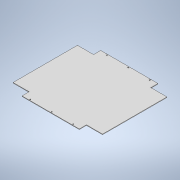
# Autodesk Inventor part: basePlate
Saved by Autodesk Inventor 2020 (Build 240168000, 168)
## iProperties
Created: 2019-06-20
Part Number: basePlate
Material: Generic
Document SubType Name: Modeling
Designer: Vivek Muskan
Density: 1 g/cm^3
Appearance: Default
Author: Vivek Muskan
Autodesk Inventor part; units mm, degrees
ref_plane "YZ Plane" through (0, 0, 0) normal (1, 0, 0) x (0, 1, 0)
ref_plane "XZ Plane" through (0, 0, 0) normal (0, 1, 0) x (-1, 0, 0)
ref_plane "XY Plane" through (0, 0, 0) normal (0, 0, 1) x (1, 0, 0)
sketch "Sketch1" plane through (0, 0, 0) normal (0, 1, 0) x (-1, 0, 0)
  line L0 (125, 90) -> (-125, 90)
  line L1 (-125, 90) -> (-125, -90)
  line L2 (-125, -90) -> (125, -90)
  line L3 (125, -90) -> (125, 90)
  line L4 (125, 90) -> (-125, -90) construction
  line L5 (-125, 90) -> (125, -90) construction
  line L6 (0, 90) -> (80, 90)
  line L7 (80, 90) -> (-80, 90)
  line L8 (-80, 90) -> (-80, 110)
  line L9 (-80, 110) -> (80, 110)
  line L10 (80, 110) -> (80, 90)
  line L11 (80, -90) -> (-80, -90)
  line L12 (-80, -90) -> (-80, -110)
  line L13 (-80, -110) -> (80, -110)
  line L14 (80, -110) -> (80, -90)
  line L15 (0, 0) -> (0, -104)
  line L16 (0, -104) -> (0, -107)
  circle A0 centre (0, -107) radius 1.5
  line L17 (0, -107) -> (60, -107)
  line L18 (0, -107) -> (-60, -107)
  circle A1 centre (60, -107) radius 1.5
  circle A2 centre (-60, -107) radius 1.5
  line L19 (0, 0) -> (20.0042, 0)
  circle A3 centre (0, 107) radius 1.5
  circle A4 centre (60, 107) radius 1.5
  circle A5 centre (-60, 107) radius 1.5
  dimension "d0" = 250
  dimension "d1" = 180
  dimension "d2" = 80
  dimension "d3" = 160
  dimension "d4" = 20
  dimension "d5" = 160
  dimension "d6" = 20
  dimension "d7" = 104
  dimension "d8" = 3
  dimension "d9" = 3
  dimension "d10" = 60
  dimension "d11" = 60
  dimension "d12" = 3
  dimension "d13" = 3
  constraints: 40 end point, 7 parallel, 6 centre point, 5 horizontal, 3 coincident, 3 midpoint, 3 perpendicular, 3 point on line, 3 symmetric about line, 1 vertical, 3 other
  measures "d0" distance of L2.end L1.end
  measures "d1" distance of L2.end L0.start
  measures "d2" distance of L6.start L6.end
  measures "d3" distance of L8.end L9.end
  measures "d4" distance of L7.end L8.end
  measures "d5" distance of L13.end L12.end
  measures "d6" distance of L12.end L11.end
  measures "d7" distance of L15.start L15.end
  measures "d8" distance of L15.end L16.end
  measures "d9" diameter of A0
  measures "d10" distance of L17.start L17.end
  measures "d11" distance of L17.start L18.end
  measures "d12" diameter of A1
  measures "d13" diameter of A2
extrude "Extrusion1" add sketch "Sketch1" along normal blind 1.5
body "Solid1"
